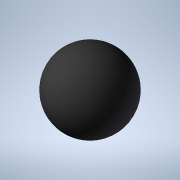
# Autodesk Inventor part: hpc_Q2307-ACC_3
Saved by Autodesk Inventor 2021 (Build 250183000, 183)
## iProperties
Created: 2026-05-26
Part Number: hpc_Q2307-ACC_3
Material: Generic
Catalog Web Link: www.3dfindit.com
Description: Q1Q2-3-Roulement à rotule sur billes - acier
Vendor: HPC
Document SubType Name: Modeling
Designer: psAdmin
Manufacturer: HPC
Mass: 1.36942 g
Surface Area: 5.9636 cm^2
Volume: 1.36942 cm^3
Density: 1 g/cm^3
Appearance: PSOLRGB-176-176-176
Category: PARTsolutions
Company: HPC
Title: HPC - Q2307-ACC
Author: Cadenas PARTsolutions
Comments: Roulement à rotule sur billes - acier
PSOL_IDENT_0: {$CADENAS_DATA/23d-libs/hpc/v3/rotary/radial/steel/q1q2/q1q2_3.prj},171 {VTYP=3D},{NB=hpc_Q2307-ACC_
PSOL_IDENT_1: 3},{LINA=HPC - Q2307-ACC},{NN=Q1Q2-3},{DATE=26.05.2021 13:15:38},{GEOMDATE=24.09.2019 07:57:00},{VER
PSOL_IDENT_2: SION=},{LINEID=220},{WBVAR=},{WBNUMERIC=}  {NB=hpc_Q2307-ACC_3},{LINA=HPC - Q2307-ACC},{KT=DUMMY},{R
PSOL_IDENT_3: EF=Q2307-ACC},{D=35},{D1=80},{B=31},{CD=38.91},{CS=10.98},{VLG=9180},{VLH=10800},{MAS=0.680},{INFO=I
PSOL_IDENT_4: NFO}
NB: hpc_Q2307-ACC_3
NN: Q1Q2-3
NT: Roulement à rotule sur billes - acier
NBSYN: hpc_$REF._3
LINA: HPC - Q2307-ACC
CATALOG: HPC
REF: Q2307-ACC
D: 35
D1: 80
B: 31
CD: 38.91
CS: 10.98
VLG: 9180
VLH: 10800
MAS: 0.68
INFO: INFO
SUPPLIER: HPC
ARTICLENO: hpc_Q2307-ACC_3
BOMINFO: HPC - Q2307-ACC
CREATOR: CADENAS GmbH
Autodesk Inventor part; units mm, degrees
sketch "Sketch_1" plane through (0, 0, 0) normal (0, 0, 1) x (1, 0, 0)
  line L0 (50, 0) -> (-50, 0)
  arc A0 (6.8889, 0) -> (-6.8889, 0) centre (0, 0) ccw
  line L1 (6.8889, 0) -> (-6.8889, 0)
  constraints: 4 end point, 2 point on circle, 1 centre point
revolve "Revolution1" add sketch "Sketch_1" angle 360 about axis through (50, 0, 0) along (1, 0, 0)
ref_plane "IP_3_XY" through (0, 0, 0) normal (1, 0, 0) x (0, 0, -1)
ref_plane "IP_3_YZ" through (0, 0, 0) normal (0, 0, -1) x (0, 1, 0)
ref_plane "IP_3_ZX" through (0, 0, 0) normal (0, 1, 0) x (1, 0, 0)
body "Solid1"
